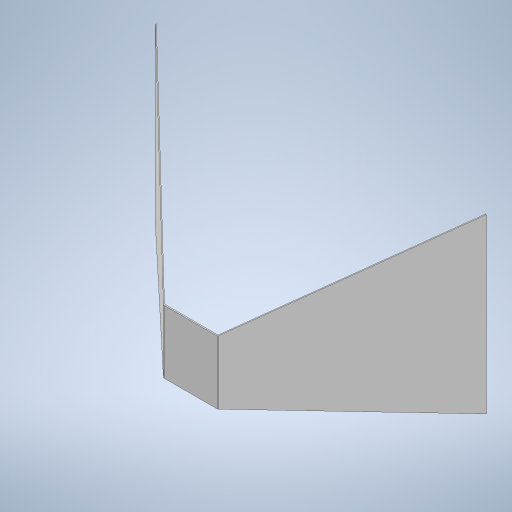
# Autodesk Inventor part: МОО 042 лист брюхо-горло
Saved by Autodesk Inventor 2024.2 (Build 282272000, 272)
## iProperties
Created: 2024-04-28
Part Number: МОО 042 лист брюхо-горло
Material: Stainless Steel
Document SubType Name: Sheet Metal
Designer: admin
Mass: 43226.5 g
Surface Area: 36190.2 cm^2
Volume: 5403.32 cm^3
Density: 8 g/cm^3
Flat Pattern Width: 71.642 cm
Flat Pattern Length: 180.083 cm
Flat Pattern Area: 12901.5 cm^2
Sheet Metal Rule: Default_mm
Sheet Metal Width: 716,420 mm
Sheet Metal Length: 1800,834 mm
Sheet Metal Area: 1290153,397 mm^2
Appearance: Default
Stock Number: МОО 042 лист брюхо-горло
Author: admin
Autodesk Inventor part; units mm, degrees
ref_plane "YZ Plane" through (0, 0, 0) normal (1, 0, 0) x (0, 1, 0)
sketch "Sketch1" plane through (0, 0, 0) normal (0, 0, 1) x (1, 0, 0)
  line L0 (-750, 0) -> (750, 0) construction
  line L1 (750, 0) -> (750, -2700) construction
  line L2 (750, -2700) -> (-750, -2700) construction
  line L3 (-750, -2700) -> (-750, 0) construction
  line L4 (800, 50) -> (-800, 50) construction
  line L5 (-800, 50) -> (-800, -2750) construction
  line L6 (-800, -2750) -> (800, -2750) construction
  line L7 (800, -2750) -> (800, 50) construction
  line L8 (-850, 100) -> (850, 100) construction
  line L9 (850, 100) -> (850, -2800) construction
  line L10 (850, -2800) -> (-850, -2800) construction
  line L11 (-850, -2800) -> (-850, 100) construction
  arc A0 (750, 0) -> (745.2706, 0.6314) centre (0, -5600) ccw construction
  line L12 (-750, -2100) -> (750, -2100) construction
  line L13 (114.1118, -2698.3696) -> (687.3692, -2158.9354)
  arc A1 (750, -2100) -> (768.2917, -213.4901) centre (-10250, -1050) ccw construction
  line L14 (750, 0) -> (749.6018, -2.9735) construction
  arc A2 (750, -3.0268) -> (0, 47) centre (-0.2, -5603) ccw construction
  line L15 (750, 0) -> (747.0136, -0.2851) construction
  arc A3 (767.1641, -238.6409) -> (747.4657, -5.0326) centre (-10252.9895, -1050.2527) ccw construction
  arc A4 (750.4522, -4.7486) -> (745.2706, 0.6314) centre (744.4791, -5.3162) ccw construction
  arc A5 (747.4657, -5.0326) -> (744.8748, -2.3426) centre (744.4792, -5.3164) ccw construction
  line L16 (750, -2100) -> (752.9864, -2100.2851) construction
  arc A6 (752.9864, -2100.2851) -> (771.2831, -213.263) centre (-10246.9891, -1050.0292) ccw construction
  line L17 (750, -2100) -> (752.0559, -2102.1848) construction
  line L18 (752.0559, -2102.1848) -> (752.0559, -2102.1848) construction
  arc A7 (749.1768, -2100.7746) -> (750.1074, -2098.8746) centre (747.1209, -2098.5898) ccw construction
  line L19 (0, -2697) -> (110, -2697) construction
  line L20 (112.0559, -2696.1848) -> (685.3133, -2156.7506) construction
  arc A8 (110, -2700) -> (114.1118, -2698.3696) centre (110, -2694) ccw
  arc A9 (110, -2697) -> (112.0559, -2696.1848) centre (110, -2694) ccw construction
  line L21 (685.3133, -2156.7506) -> (687.3692, -2158.9354) construction
  line L22 (752.0559, -2102.1848) -> (671.2185, -2178.2526) construction
  line L23 (671.2185, -2178.2526) -> (669.1626, -2176.0678) construction
  arc A10 (747.4657, -5.0326) -> (747.0136, -0.2851) centre (-10252.9895, -1050.2527) ccw construction
  arc A11 (745.2706, 0.6314) -> (0, 50) centre (0, -5600) ccw construction
  arc A12 (750.4522, -4.7486) -> (750, 0) centre (-10250, -1050) ccw construction
  line L24 (770.156, -238.4205) -> (767.1641, -238.6409) construction
  line L25 (768.2917, -213.4901) -> (771.2831, -213.263) construction
  arc A13 (768.2917, -213.4901) -> (750.4522, -4.7486) centre (-10250, -1050) ccw construction
  line L26 (0, 100) -> (0, 50) construction
  line L27 (0, -2700) -> (0, -2697) construction
  line L28 (0, 47) -> (0, 0) construction
  line L29 (0, 50) -> (0, 47) construction
  arc A14 (752.0559, -2102.1848) -> (752.9864, -2100.2851) centre (749.9983, -2099.9992) ccw construction
  line L30 (0, -2700) -> (110, -2700)
  line L31 (687.3692, -2158.9354) -> (750, -2100) construction
  point P0 (0, -2750)
  dimension "d19" = 1500
  dimension "d20" = 2700
  dimension "d21" = 2100
  dimension "d22" = 6
  dimension "d23" = 3
  dimension "d24" = 3
  dimension "d25" = 6
  dimension "d26" = 3
  dimension "d27" = 239.271
  dimension "d28" = 50
  dimension "d29" = 50
  dimension "d30" = 3
  dimension "d31" = 25
  dimension "d32" = 110
  dimension "d33" = 25
  dimension "d34" = 111
  measures "d19" distance of L3.end L1.start
  measures "d20" distance of L1.start L2.start
  measures "d21" distance between parallel lines of L12 L0
  measures "d22" radius of A4
  measures "d23" radius of A5
  measures "d24" radius of A7
  measures "d25" radius of A8
  measures "d26" radius of A9
  measures "d27" distance of L1.start L24.start
  measures "d28" distance between parallel lines of L4 L8
  measures "d29" distance between parallel lines of L0 L4
  measures "d30" distance of L29.start L29.end
  measures "d31" distance of L24.start L25.start
  measures "d32" distance from line of L27 A8.centre
  measures "d33" distance of L23.end L13.end
  measures "d34" distance of L12.end L23.end
contour flange "Contour Flange1" sketch "Sketch1" thickness 3 bend radius 3 width 1240 along (0, 0, 1) mid plane no both sides no wall seen from (55, -2700, 0) lies toward (0, 1, 0) curves L30 A8 L13
bend "Bend1"
corner "Corner1"
mirror "Mirror1" about plane through (0, 0, 0) normal (1, 0, 0)
sketch "Sketch2" plane through (0, 0, 0) normal (1, 0, 0) x (0, 1, 0)
  line L0 (-2700, 1240) -> (-2700, 0) projected
  line L1 (-2700, 1240) -> (-2700, 0) projected
  line L2 (-2156.7506, 0) -> (-2156.7506, 1240) projected
  line L3 (-2156.7506, 0) -> (-2156.7506, 1240) projected
  line L4 (-2156.7506, 1240) -> (-2700, 1240)
  line L5 (-2156.7506, 717.8371) -> (-2700, 261.9968)
  point P0 (0, 0)
  dimension "d46" = 40
  dimension "d64" = 261.9968
  dimension "d66" = 400
  constraints: 4 end point, 2 point on line
  measures "d46" angle of L5 L4
  measures "d64" distance of L0.end L5.end
  measures "d66" distance from line of L5 L2.end
extrude "Extrusion1" cut sketch "Sketch2" along normal through all both and the other way through all
ref_plane "Work Plane1" through (-110, -2378.6062, -121.0255) normal (0, -0.6427876, 0.7660444) x (1, 0, 0)
sketch "Sketch3" plane through (-110, -2378.6062, -121.0255) normal (0, -0.6427876, 0.7660444) x (1, 0, 0)
  line L0 (110, 832.5917) -> (110, -167.4083)
  line L1 (110, 832.5917) -> (150, 832.5917)
  line L2 (150, 832.5917) -> (150, -167.4083)
  line L3 (150, -167.4083) -> (110, -167.4083)
  line L4 (0, -168.4083) -> (220, -168.4083) projected
  point P0 (110, 1899.9117)
  point P1 (110, -168.4083)
  dimension "d50" = 80
  dimension "d51" = 1000
  dimension "d53" = 1
  dimension "d55" = 0
  constraints: 8 end point, 2 perpendicular, 1 horizontal, 1 midpoint, 1 vertical
  measures "d50" diameter of L2 L0
  measures "d51" distance of L1.end L2.end
  measures "d53" distance between parallel lines of L4 L3
  measures "d55" distance from line of point (110, -168.408) L0
revolve "Revolution1" [suppressed]
fillet "Fillet1" radius 2 2 edges at (686.3413, -2157.843, 716.9205) (-686.3413, -2157.843, 716.9205)
ref_plane "Work Plane2" through (-110, -2571.4425, 108.7879) normal (0, -0.6427876, 0.7660444) x (1, 0, 0)
sketch "Sketch5" plane through (-110, -2571.4425, 108.7879) normal (0, -0.6427876, 0.7660444) x (1, 0, 0)
  line L0 (0, -168.4083) -> (220, -168.4083) projected
  line L1 (510, -168.4083) -> (510, 706.5844)
  line L2 (510, 706.5844) -> (595, 706.5844)
  line L3 (595, 706.5844) -> (595, -168.4083)
  line L4 (595, -168.4083) -> (510, -168.4083)
  point P0 (110, 1899.9117)
  point P1 (793.2152, 706.5844)
  point P2 (110, -168.4083)
  dimension "d61" = 170
  dimension "d62" = 400
  constraints: 8 end point, 2 horizontal alignment, 2 perpendicular, 1 horizontal, 1 midpoint, 1 vertical
  measures "d61" diameter of L3 L1
  measures "d62" distance of point (110, -168.408) L1.start
revolve "Revolution2" [suppressed]
mirror "Mirror2" [suppressed]
equation "\"d19\" = Бак_ширина_общая"
equation "\"d20\" = Бак_высота_общая"
equation "\"d21\" = Бак_высота_до_конуса"
equation "\"d22\" = Thickness + BendRadius"
equation "\"d23\" = Thickness"
equation "\"d24\" = Thickness"
equation "\"d25\" = Thickness + BendRadius"
equation "\"d26\" = Thickness"
equation "\"d27\" = Бак_спина_длина_фланцев"
equation "\"d30\" = d40"
equation "\"d31\" = Бак_нахлест_фланца"
equation "\"d32\" = 0.5 * Бак_брюхо_ширина_полки"
equation "\"d33\" = Бак_нахлест_фланца"
equation "\"d34\" = Бак_борт_длина_фланца"
equation "\"d7\" = Thickness"
equation "\"d8\" = BendReliefWidth"
equation "\"d9\" = BendReliefDepth"
equation "\"d10\" = MinimumRemnant"
equation "\"d11\" = TransitionRadius"
equation "\"d13\" = BendRadius"
equation "\"d15\" = CornerReliefSize"
equation "\"d16\" = GapSize"
equation "\"d17\" = JacobiRadiusSize"
equation "\"BendRadius\" = Thickness"
equation "\"BendReliefWidth\" = Thickness"
equation "\"BendReliefDepth\" = 0.5 * Thickness"
equation "\"CornerReliefSize\" = 4 * Thickness"
equation "\"MinimumRemnant\" = 2 * Thickness"
equation "\"TransitionRadius\" = BendRadius"
equation "\"JacobiRadiusSize\" = BendRadius"
equation "\"GapSize\" = Thickness"
equation "\"d38\" = d40 + d44"
equation "\"d39\" = d40"
equation "\"d44\" = d40"
equation "\"Бак_ширина_общая\" = 1500"
equation "\"Бак_высота_общая\" = 2700"
equation "\"Бак_высота_до_конуса\" = 2100"
equation "\"Thickness\" = 3"
equation "\"Бак_спина_длина_фланцев\" = 239.271"
equation "\"d40\" = 3"
equation "\"Бак_нахлест_фланца\" = 25"
equation "\"Бак_брюхо_ширина_полки\" = 220"
equation "\"Бак_борт_длина_фланца\" = 111"
body "Solid1"
